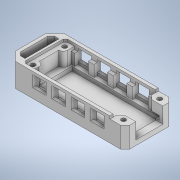
# Autodesk Inventor part: Case_main
Saved by Autodesk Inventor 2020 (Build 240168000, 168)
## iProperties
Created: 2022-03-19
Part Number: Case_main
Material: Типовые
Document SubType Name: Modeling
Designer: NoName
Density: 1 g/cm^3
Appearance: По умолчанию
Author: NoName
Autodesk Inventor part; units mm, degrees
ref_plane "YZ Plane" through (0, 0, 0) normal (1, 0, 0) x (0, 1, 0)
ref_plane "XZ Plane" through (0, 0, 0) normal (0, 1, 0) x (-1, 0, 0)
sketch "Эскиз1" plane through (0, 0, 0) normal (0, 1, 0) x (-1, 0, 0)
  line L0 (0, 0) -> (0, -18.6)
  line L1 (0, -18.6) -> (40.8, -18.6)
  line L2 (40.8, -18.6) -> (40.8, -15.65)
  arc A0 (42.8, -13.65) -> (40.8, -15.65) centre (42.8, -15.65) ccw
  line L3 (42.8, -15.65) -> (42.8, -13.65) construction
  line L4 (42.8, -15.65) -> (40.8, -15.65) construction
  line L5 (42.8, -13.65) -> (42.8, -4.95)
  line L6 (42.8, -9.3) -> (0, -9.3)
  line L7 (0, 0) -> (40.8, 0)
  line L8 (40.8, 0) -> (40.8, -2.95)
  arc A1 (40.8, -2.95) -> (42.8, -4.95) centre (42.8, -2.95) ccw
  line L9 (42.8, -2.95) -> (42.8, -4.95) construction
  line L10 (42.8, -2.95) -> (40.8, -2.95) construction
  line L11 (46.8, -20) -> (0.4, -20)
  line L12 (46.8, 1.4) -> (0.4, 1.4)
  line L13 (50.8, -16) -> (50.8, -2.6)
  line L14 (45.8, -16.8) -> (45.8, -1.8)
  line L15 (49.3, -15.3787) -> (49.3, -3.2213)
  line L16 (5.1, -18.6) -> (5.1, -17.2)
  line L17 (5.1, -17.2) -> (0, -17.2)
  line L18 (5.1, 0) -> (5.1, -1.4)
  line L19 (5.1, -1.4) -> (0, -1.4)
  line L20 (0.4, -20) -> (-1.6, -18)
  line L21 (-1.6, -18) -> (-1.6, -0.6)
  line L22 (-1.6, -0.6) -> (0.4, 1.4)
  line L23 (46.8, 1.4) -> (50.8, -2.6)
  line L24 (50.8, -16) -> (46.8, -20)
  line L25 (49.3, -15.3787) -> (47.8787, -16.8)
  line L26 (47.8787, -16.8) -> (45.8, -16.8)
  line L27 (49.3, -3.2213) -> (47.8787, -1.8)
  line L28 (47.8787, -1.8) -> (45.8, -1.8)
  point P0 (5.1, 0)
  point P1 (0, -1.4)
  point P2 (45.8, -9.3)
  point P3 (49.3, -9.3)
  point P4 (50.8, -9.3)
  dimension "d1" = 42.8
  dimension "d3" = 2
  dimension "d4" = 12.7
  dimension "d8" = 18.6
  dimension "d12" = 3.5
  dimension "d32" = 21.4
  dimension "d34" = 5.1
  dimension "d35" = 15.8
  dimension "d41" = 135
  dimension "d42" = 1.6
  dimension "d43" = 2
  dimension "d65" = 8
  dimension "d66" = 1.5
  dimension "d67" = 15
  dimension "d68" = 1.5
  dimension "d69" = 4
  constraints: 59 end point, 13 symmetric about line, 7 vertical, 6 perpendicular, 5 midpoint, 4 point on circle, 3 horizontal alignment, 2 centre point, 2 point on line, 1 horizontal, 1 parallel, 1 tangent, 1 other
  measures "d1" distance between parallel lines of L0 L5
  measures "d3" distance between parallel lines of L5 L8
  measures "d4" distance of L9.start L3.start
  measures "d8" distance between parallel lines of L7 L1
  measures "d12" distance between parallel lines of L15 L14
  measures "d32" distance between parallel lines of L12 L11
  measures "d34" distance between parallel lines of L0 L16
  measures "d35" distance between parallel lines of L19 L17
  measures "d41" angle of L12 L22
  measures "d42" distance between parallel lines of L0 L21
  measures "d43" horizontal distance of L21.end L12.end
  measures "d65" distance between parallel lines of L5 L13
  measures "d66" distance between parallel lines of L13 L15
  measures "d67" distance between parallel lines of L28 L26
  measures "d68" distance between parallel lines of L24 L25
  measures "d69" distance from line of L5 L11.start
extrude "Выдавливание1" add sketch "Эскиз1" along normal blind 6.2 contours L7 L18 L19 L0 | L17 L16 L1 L0 | L11 L20 L21 L22 L12 L23 L13 L24
sketch "Эскиз2" plane through (0, 0, 0) normal (0, -1, 0) x (1, 0, 0)
  line L0 (-0.4, -20) -> (-46.8, -20) projected
  line L1 (-46.8, 1.4) -> (-0.4, 1.4) projected
  line L2 (-50.8, -16) -> (-50.8, -2.6) projected
  line L3 (-42.8, -4.95) -> (-42.8, -13.65) projected
  arc A0 (-42.8, -4.95) -> (-40.8, -2.95) centre (-42.8, -2.95) ccw projected
  line L4 (-40.8, 0) -> (-40.8, -2.95) projected
  line L5 (-5.1, 0) -> (-40.8, 0) projected
  line L6 (0, -17.2) -> (0, -1.4) projected
  line L7 (-40.8, -18.6) -> (-5.1, -18.6) projected
  line L8 (-40.8, -15.65) -> (-40.8, -18.6) projected
  arc A1 (-40.8, -15.65) -> (-42.8, -13.65) centre (-42.8, -15.65) ccw projected
  line L9 (-40.8, -15.65) -> (-40.8, -18.6) projected
  line L10 (-40.8, -18.6) -> (-5.1, -18.6) projected
  line L11 (-39.8, -16.6) -> (-1.5, -16.6)
  line L12 (-1.5, -16.6) -> (-1.5, -2)
  line L13 (-1.5, -2) -> (-39.8, -2)
  line L14 (-39.8, -2) -> (-39.8, -16.6)
  line L15 (-5.1, -1.4) -> (-5.1, 0) projected
  line L16 (0, -1.4) -> (-5.1, -1.4) projected
  line L17 (-5.1, -17.2) -> (0, -17.2) projected
  line L18 (-5.1, -18.6) -> (-5.1, -17.2) projected
  line L19 (1.6, -18) -> (-0.4, -20) projected
  line L20 (1.6, -0.6) -> (1.6, -18) projected
  line L21 (-0.4, 1.4) -> (1.6, -0.6) projected
  line L22 (-50.8, -2.6) -> (-46.8, 1.4) projected
  line L23 (-46.8, -20) -> (-50.8, -16) projected
  line L24 (-49.3, -3.2213) -> (-49.3, -15.3787) projected
  line L25 (-47.8787, -1.8) -> (-49.3, -3.2213) projected
  line L26 (-45.8, -1.8) -> (-47.8787, -1.8) projected
  line L27 (-45.8, -16.8) -> (-45.8, -1.8) projected
  line L28 (-47.8787, -16.8) -> (-45.8, -16.8) projected
  line L29 (-49.3, -15.3787) -> (-47.8787, -16.8) projected
  point P0 (0, -18.2)
  point P1 (-42.8, -9.3)
  point P2 (-39.8, -9.3)
  dimension "d17" = 1.5
  dimension "d18" = 3
  dimension "d33" = 14.6
  constraints: 8 end point, 2 midpoint, 2 parallel, 1 horizontal, 1 horizontal alignment, 1 perpendicular, 1 other
  measures "d17" distance between parallel lines of L6 L12
  measures "d18" distance between parallel lines of L3 L14
  measures "d33" distance between parallel lines of L13 L11
extrude "Выдавливание2" add sketch "Эскиз2" along normal blind 1.8 contours L0 L23 L2 L22 L1 L21 L20 L19 | A0 L4 L5 L15 L16 L6 L17 L18 L7 L8 A1 L3
sketch "Эскиз3" plane through (0, -1.8, 0) normal (0, -1, 0) x (1, 0, 0)
  line L0 (-0.4, 1.4) -> (-46.8, 1.4) projected
  line L1 (-50.8, -2.6) -> (-50.8, -16) projected
  line L2 (-46.8, -20) -> (-0.4, -20) projected
  line L3 (-1.5, -2) -> (-1.5, -16.6) projected
  line L4 (-1.5, -16.6) -> (-39.8, -16.6) projected
  line L5 (-39.8, -16.6) -> (-39.8, -2) projected
  line L6 (-39.8, -2) -> (-1.5, -2) projected
  line L7 (-0.4, -20) -> (1.6, -18) projected
  line L8 (1.6, -18) -> (1.6, -0.6) projected
  line L9 (1.6, -0.6) -> (-0.4, 1.4) projected
  line L10 (-46.8, 1.4) -> (-50.8, -2.6) projected
  line L11 (-50.8, -16) -> (-46.8, -20) projected
  line L12 (-49.3, -15.3787) -> (-49.3, -3.2213) projected
  line L13 (-49.3, -3.2213) -> (-47.8787, -1.8) projected
  line L14 (-47.8787, -1.8) -> (-45.8, -1.8) projected
  line L15 (-45.8, -1.8) -> (-45.8, -16.8) projected
  line L16 (-45.8, -16.8) -> (-47.8787, -16.8) projected
  line L17 (-47.8787, -16.8) -> (-49.3, -15.3787) projected
  point P0 (0, 0)
extrude "Выдавливание3" add sketch "Эскиз3" along normal blind 1.2 contours L9 L8 L7 L2 L11 L1 L10 L0 | L3 L4 L5 L6
sketch "Эскиз5" plane through (-46.8, 6.2, 1.4) normal (0, 0, 1) x (1, 0, 0)
  line L0 (7.6, 0) -> (13.6, 0)
  line L1 (13.6, 0) -> (13.6, -5)
  line L2 (13.6, -5) -> (7.6, -5)
  line L3 (7.6, -5) -> (7.6, 0)
  line L4 (0, 0) -> (46.4, 0) projected
  line L5 (4, -6.2) -> (4, 0) projected
  point P0 (46.8, -6.2)
  point P1 (46.5, 0)
  dimension "d27" = 6
  dimension "d28" = 5
  dimension "d29" = 3.6
  constraints: 8 end point, 2 parallel, 1 horizontal, 1 perpendicular, 1 point on line
  measures "d27" distance between parallel lines of L3 L1
  measures "d28" distance between parallel lines of L0 L2
  measures "d29" distance between parallel lines of L5 L3
extrude "Выдавливание5" cut sketch "Эскиз5" against normal through all
pattern_linear "Прямоуг.массив1" count 4 spacing 8.5 along (1, 0, 0) of "Выдавливание5"
sketch "Эскиз6" plane through (0, 0, 0) normal (0, 1, 0) x (1, 0, 0)
  line L0 (-5.1, 0) -> (-40.8, 0) projected
  line L1 (-16.2, 0) -> (-13.7, 0)
  line L2 (-13.7, 0) -> (-13.7, 1.4)
  line L3 (-13.7, 1.4) -> (-16.2, 1.4)
  line L4 (-16.2, 1.4) -> (-16.2, 0)
  line L5 (-24.7, 0) -> (-22.2, 0)
  line L6 (-22.2, 0) -> (-22.2, 1.4)
  line L7 (-22.2, 1.4) -> (-24.7, 1.4)
  line L8 (-24.7, 1.4) -> (-24.7, 0)
  line L9 (-33.2, 0) -> (-30.7, 0)
  line L10 (-30.7, 0) -> (-30.7, 1.4)
  line L11 (-30.7, 1.4) -> (-33.2, 1.4)
  line L12 (-33.2, 1.4) -> (-33.2, 0)
  line L13 (-39.2, 0) -> (-40.8, 0)
  line L14 (-40.8, 0) -> (-40.8, 1.4)
  line L15 (-40.8, 1.4) -> (-39.2, 1.4)
  line L16 (-39.2, 1.4) -> (-39.2, 0)
  line L17 (-5.1, 0) -> (-7.7, 0) projected
  line L18 (-5.1, 0) -> (-40.8, 0) projected
  line L19 (-39.2, 0) -> (-40.8, 0) projected
  line L20 (-39.2, 0) -> (-33.2, 0) projected
  line L21 (0, 1.4) -> (-5.1, 1.4) projected
  line L22 (-6.7, 0) -> (-5.1, 0)
  line L23 (-5.1, 0) -> (-5.1, 1.4)
  line L24 (-5.1, 1.4) -> (-6.7, 1.4)
  line L25 (-6.7, 1.4) -> (-6.7, 0)
  line L26 (-42.8, 4.95) -> (-42.8, 13.65) projected
  line L27 (-42.8, 9.3) -> (-1.5, 9.3)
  line L28 (-5.1, 18.6) -> (-40.8, 18.6)
  line L29 (-16.2, 18.6) -> (-13.7, 18.6)
  line L30 (-13.7, 18.6) -> (-13.7, 17.2)
  line L31 (-13.7, 17.2) -> (-16.2, 17.2)
  line L32 (-16.2, 17.2) -> (-16.2, 18.6)
  line L33 (-24.7, 18.6) -> (-22.2, 18.6)
  line L34 (-22.2, 18.6) -> (-22.2, 17.2)
  line L35 (-22.2, 17.2) -> (-24.7, 17.2)
  line L36 (-24.7, 17.2) -> (-24.7, 18.6)
  line L37 (-33.2, 18.6) -> (-30.7, 18.6)
  line L38 (-30.7, 18.6) -> (-30.7, 17.2)
  line L39 (-30.7, 17.2) -> (-33.2, 17.2)
  line L40 (-33.2, 17.2) -> (-33.2, 18.6)
  line L41 (-39.2, 18.6) -> (-40.8, 18.6)
  line L42 (-40.8, 18.6) -> (-40.8, 17.2)
  line L43 (-40.8, 17.2) -> (-39.2, 17.2)
  line L44 (-39.2, 17.2) -> (-39.2, 18.6)
  line L45 (-5.1, 18.6) -> (-6.7, 18.6)
  line L46 (-5.1, 18.6) -> (-40.8, 18.6)
  line L47 (-39.2, 18.6) -> (-40.8, 18.6)
  line L48 (-39.2, 18.6) -> (-33.2, 18.6)
  line L49 (-30.7, 18.6) -> (-33.2, 18.6)
  line L50 (-30.7, 18.6) -> (-24.7, 18.6)
  line L51 (-22.2, 18.6) -> (-24.7, 18.6)
  line L52 (-22.2, 18.6) -> (-16.2, 18.6)
  line L53 (-13.7, 18.6) -> (-16.2, 18.6)
  line L54 (-12.7, 18.4) -> (-6.7, 18.4)
  line L55 (0, 17.2) -> (-5.1, 17.2)
  line L56 (-6.7, 18.6) -> (-5.1, 18.6)
  line L57 (-5.1, 18.6) -> (-5.1, 17.2)
  line L58 (-5.1, 17.2) -> (-6.7, 17.2)
  line L59 (-6.7, 17.2) -> (-6.7, 18.6)
  line L60 (-1.5, 2) -> (-1.5, 16.6) projected
  line L61 (-30.7, 0) -> (-33.2, 0) projected
  line L62 (-30.7, 0) -> (-24.7, 0) projected
  line L63 (-22.2, 0) -> (-24.7, 0) projected
  line L64 (-22.2, 0) -> (-16.2, 0) projected
  line L65 (-13.7, 0) -> (-16.2, 0) projected
  line L66 (-13.7, 0) -> (-7.7, 0) projected
  point P0 (0, 0)
  point P1 (0, 18.6)
  point P2 (-22.2, 18.6)
  point P3 (-6.7, 0)
  point P4 (-13.7, 0)
  point P5 (-22.2, 0)
  point P6 (-30.7, 0)
  constraints: 106 end point, 29 symmetric about line, 10 parallel, 10 point on line, 6 horizontal, 5 perpendicular, 4 horizontal alignment, 2 midpoint
extrude "Выдавливание6" add sketch "Эскиз6" along normal blind 5
sketch "Эскиз7" plane through (1.6, 6.2, -0.6) normal (1, 0, 0) x (0, 0, -1)
  line L0 (16.2, 0) -> (1.2, 0) projected
  line L1 (14.7, 0) -> (2.7, 0)
  line L2 (2.7, 0) -> (2.7, -7)
  line L3 (2.7, -7) -> (14.7, -7)
  line L4 (14.7, -7) -> (14.7, 0)
  point P0 (-0.6, -6.2)
  point P1 (16.5, 0)
  point P2 (-0.5, 0)
  point P3 (8.7, 0)
  point P4 (2.7, 0)
  dimension "d44" = 12
  dimension "d45" = 7
  constraints: 8 end point, 2 midpoint, 2 parallel, 1 horizontal, 1 perpendicular, 1 point on line
  measures "d44" distance between parallel lines of L4 L2
  measures "d45" distance between parallel lines of L3 L0
extrude "Выдавливание7" cut sketch "Эскиз7" against normal up to next
ref_plane "РабПлоскость1" through (0, 1.8, 0) normal (0, 1, 0) x (1, 0, 0)
sketch "Эскиз8" plane through (0, 1.8, 0) normal (0, 1, 0) x (1, 0, 0)
  line L0 (0, 17.2) -> (0, 15.3) projected
  line L1 (0, 17.2) -> (-5.1, 17.2)
  line L2 (0, 15.3) -> (0, 17.2)
  line L3 (-42.8, 4.95) -> (-42.8, 13.65) projected
  line L4 (-42.8, 9.3) -> (1.6, 9.3)
  line L5 (1.6, 15.3) -> (1.6, 3.3) projected
  line L6 (-5.1, 17.2) -> (-3.2, 15.3)
  line L7 (-3.2, 15.3) -> (0, 15.3)
  line L8 (0, 17.2) -> (-6.7, 17.2) projected
  line L9 (0, 1.4) -> (0, 3.3)
  line L10 (0, 1.4) -> (-5.1, 1.4)
  line L11 (0, 3.3) -> (0, 1.4)
  line L12 (-5.1, 1.4) -> (-3.2, 3.3)
  line L13 (-3.2, 3.3) -> (0, 3.3)
  point P0 (0, 0)
  point P1 (-6.7, 17.1)
  point P2 (-6.7, 17.2)
  dimension "d49" = 45
  constraints: 20 end point, 5 symmetric about line, 2 horizontal, 2 midpoint, 2 point on line, 1 other
  measures "d49" angle of L1 L6
extrude "Выдавливание8" add sketch "Эскиз8" along normal up to surface (4.4 mm away)
sketch "Эскиз10" plane through (0, 6.2, 0) normal (0, 1, 0) x (1, 0, 0)
  line L0 (-42.8, 4.95) -> (-42.8, 13.65) projected
  line L1 (-42.8, 9.3) -> (-1.5, 9.3)
  line L2 (-1.5, 2) -> (-1.5, 16.6) projected
  line L3 (-45.8, 16.8) -> (-45.8, 1.8) projected
  line L4 (1.6, 15.3) -> (1.6, 18) projected
  point P0 (0, 0)
  point P1 (-42.8, 16.3)
  point P2 (-42.8, 2.3)
  point P3 (-1.8, 17.3)
  point P4 (-1.8, 1.3)
  point P5 (-44.8, 17.7)
  point P6 (-44.8, 0.7)
  point P7 (-45.8, 1.8)
  dimension "d59" = 16
  dimension "d60" = 14
  dimension "d62" = 3.4
  dimension "d76" = 41
  constraints: 2 end point, 2 midpoint, 2 symmetric about line, 1 other
  measures "d59" distance of point (-1.8, 1.3) point (-1.8, 17.3)
  measures "d60" distance of point (-42.8, 2.3) point (-42.8, 16.3)
  measures "d62" distance from line of L4 point (-1.8, 17.3)
  measures "d76" horizontal distance of point (-42.8, 16.3) point (-1.8, 17.3)
hole "Отверстие1" at (-42.8, 6.2, -16.3) at (-42.8, 6.2, -2.3) at (-1.8, 6.2, -17.3) at (-1.8, 6.2, -1.3) direction (0, -1, 0) diameter 2 depth 6.2
sketch "Эскиз13" plane through (0, 6.2, 0) normal (0, 1, 0) x (1, 0, 0)
  circle A0 centre (-42.8, 16.3) radius 1 projected
  circle A1 centre (-42.8, 2.3) radius 1 projected
  line L0 (-47.8787, 1.8) -> (-49.3, 3.2213) projected
  line L1 (-49.3, 3.2213) -> (-49.3, 15.3787) projected
  line L2 (-49.3, 15.3787) -> (-47.8787, 16.8) projected
  line L3 (-47.8787, 16.8) -> (-45.8, 16.8) projected
  line L4 (-45.8, 16.8) -> (-45.8, 1.8) projected
  line L5 (-45.8, 1.8) -> (-47.8787, 1.8) projected
  line L6 (-50.8, 2.6) -> (-46.8, -1.4) projected
  line L7 (-46.8, -1.4) -> (-39.2, -1.4) projected
  line L8 (-39.2, -1.4) -> (-39.2, 0) projected
  line L9 (-39.2, 0) -> (-40.8, 0) projected
  line L10 (-40.8, 0) -> (-40.8, 2.95) projected
  arc A2 (-40.8, 2.95) -> (-42.8, 4.95) centre (-42.8, 2.95) ccw projected
  line L11 (-42.8, 4.95) -> (-42.8, 13.65) projected
  arc A3 (-42.8, 13.65) -> (-40.8, 15.65) centre (-42.8, 15.65) ccw projected
  line L12 (-40.8, 15.65) -> (-40.8, 18.6) projected
  line L13 (-40.8, 18.6) -> (-39.2, 18.6) projected
  line L14 (-39.2, 18.6) -> (-39.2, 20) projected
  line L15 (-39.2, 20) -> (-46.8, 20) projected
  line L16 (-46.8, 20) -> (-50.8, 16) projected
  line L17 (-50.8, 16) -> (-50.8, 2.6) projected
  line L18 (-40.8, 18.6) -> (-39.2, 18.6) projected
  line L19 (-7.7, 18.6) -> (-13.7, 18.6) projected
  line L20 (-39.2, 18.6) -> (-7.7, 18.6)
  line L21 (-5.1, 18.6) -> (-5.1, 17.2) projected
  line L22 (-7.7, 18.6) -> (-5.1, 18.6)
  line L23 (-5.1, 18.6) -> (-5.1, 20)
  line L24 (-0.4, 20) -> (-7.7, 20) projected
  line L25 (-5.1, 20) -> (-39.2, 20)
  line L26 (-46.8, 20) -> (-0.4, 20) projected
  line L27 (-39.2, 0) -> (-40.8, 0) projected
  line L28 (-5.1, 0) -> (-24.7, 0) projected
  line L29 (-39.2, 0) -> (-5.1, 0)
  line L30 (-5.1, 0) -> (-5.1, -1.4)
  line L31 (-0.4, -1.4) -> (-46.8, -1.4) projected
  line L32 (-39.2, -1.4) -> (-39.2, 0) projected
  line L33 (-5.1, -1.4) -> (-39.2, -1.4)
  line L34 (-40.8, 0) -> (-40.8, 1.4) projected
  line L35 (-40.8, 18.6) -> (-43.8, 18.6)
  line L36 (-43.8, 18.6) -> (-44.8, 17.6)
  line L37 (-44.8, 17.6) -> (-44.8, 1)
  line L38 (-44.8, 1) -> (-43.8, 0)
  line L39 (-43.8, 0) -> (-40.8, 0)
  line L40 (-42.8, 4.95) -> (-42.8, 13.65) projected
  line L41 (-42.8, 9.3) -> (-1.5, 9.3)
  line L42 (-1.5, 2) -> (-1.5, 16.6) projected
  point P0 (0, 0)
  point P1 (-6.7, 0)
  point P2 (-1.5, 2.1165)
  point P3 (-1.5, 16.2835)
  point P4 (-6.7, 0)
  dimension "d71" = 1
  dimension "d72" = 1
  constraints: 26 end point, 5 perpendicular, 4 horizontal, 2 collinear, 2 midpoint, 2 point on line, 1 parallel, 1 other
  measures "d71" distance between parallel lines of L4 L37
  measures "d72" horizontal distance of L35.end L36.end
extrude "Выдавливание9" add sketch "Эскиз13" along normal blind 1.2 contours L17 L16 L15 L14 L13 L35 L36 L37 L38 L39 L9 L8 L7 L6 | L8 L29 L28 L30 L31 | L25 L24 L23 L22 L19 L20 L14
